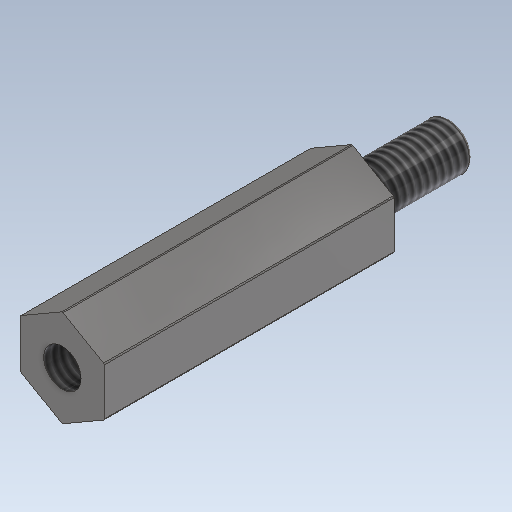
# Autodesk Inventor part: spacer
Saved by Autodesk Inventor 2020.3 (Build 243373000, 373)
## iProperties
Created: 2016-01-25
Part Number: spacer
Material: Steel, Mild
Document SubType Name: Modeling
Designer: Nanjar
Density: 7.85 g/cm^3
Appearance: Semi-Polished
Mass: 3.92973 g
Surface Area: 5.41762 cm^2
Volume: 0.500603 cm^3
Author: Nanjar
Autodesk Inventor part; units mm, degrees
ref_plane "YZ Plane" through (0, 0, 0) normal (1, 0, 0) x (0, 1, 0)
ref_plane "XZ Plane" through (0, 0, 0) normal (0, 1, 0) x (-1, 0, 0)
ref_plane "XY Plane" through (0, 0, 0) normal (0, 0, 1) x (1, 0, 0)
sketch "Sketch1" plane through (0, 0, 0) normal (0, 0, 1) x (1, 0, 0)
  line L0 (-2.75, 1.59) -> (0, 3.18)
  line L1 (0, -3.18) -> (-2.75, -1.59)
  line L2 (-2.75, 1.59) -> (-2.75, -1.59)
  line L3 (2.75, 1.59) -> (0, 3.18)
  line L4 (0, -3.18) -> (2.75, -1.59)
  line L5 (2.75, 1.59) -> (2.75, -1.59)
  point P0 (0, 0)
  constraints: 12 end point, 1 vertical
extrude "Extrusion1" add sketch "Sketch1" along normal blind 19
sketch "Sketch2" plane through (0, 0, 19) normal (0, 0, 1) x (1, 0, 0)
  circle A0 centre (0, 0) radius 1.5
  dimension "d20" = 3
  constraints: 1 centre point, 1 coincident
  measures "d20" diameter of A0
hole "Hole1" at (0, 0, 19) direction (0, 0, -1) diameter 2.459 depth 8.8 tip angle 118 thread size "M3x0.5" class "6H" standard "ISO Metric profile"
fillet "Fillet1" radius 0.1 6 edges at (0, 3.18, 9.5) (2.75, 1.59, 9.5) (-2.75, 1.59, 9.5) (2.75, -1.59, 9.5) (0, -3.18, 9.5) (-2.75, -1.59, 9.5)
sketch "Sketch4" plane through (0, 0, 0) normal (0, 0, -1) x (-1, 0, 0)
  circle A0 centre (0, 0) radius 1.5
  dimension "d29" = 3
  constraints: 1 centre point, 1 coincident
  measures "d29" diameter of A0
extrude "Extrusion2" add sketch "Sketch4" along normal blind 6.4
thread "Thread1" size "M3x0.5" class "6g" standard "ANSI Metric M Profile" length 9.967
fillet "Fillet2" radius 0.2 1 edges at (1.5, 0, -6.4)
body "Solid1"
